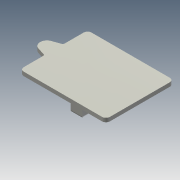
# Autodesk Inventor part: ball
Saved by Autodesk Inventor 2015 (Build 190159000, 159)
## iProperties
Created: 2017-05-03
Part Number: ball
Material: 일반
Document SubType Name: Modeling
Designer: gatew
Density: 1 g/cm^3
Appearance: 기본값
Author: gatew
Autodesk Inventor part; units mm, degrees
ref_plane "작업 평면3" through (0, 30.3443, 0) normal (0, 1, 0) x (1, 0, 0)
sketch "스케치5" plane through (0, 30.3443, 0) normal (0, 1, 0) x (1, 0, 0)
  line L0 (-35, -52.5) -> (35, -52.5)
  line L1 (35, -52.5) -> (35, 52.5)
  line L2 (35, 52.5) -> (-35, 52.5)
  line L3 (-35, 52.5) -> (-35, -52.5)
  line L4 (-35, -52.5) -> (35, 52.5) construction
  line L5 (35, -52.5) -> (-35, 52.5) construction
  point P0 (0, 0)
  dimension "d33" = 70
  dimension "d34" = 105
  constraints: 12 end point, 2 midpoint, 2 parallel, 1 horizontal, 1 perpendicular
  measures "d33" distance of L2.end L1.end
  measures "d34" distance of L1.end L0.end
extrude "돌출3" add sketch "스케치5" along normal blind 4
ref_plane "작업 평면4" through (0, 30.3443, 0) normal (0, -1, 0) x (1, 0, 0)
ref_plane "작업 평면1" through (0, 0, 0) normal (0, -0.7071068, 0.7071068) x (1, 0, 0)
ref_plane "작업 평면2" through (0, 17.1721, 0) normal (0, 1, 0) x (-1, 0, 0)
sketch "스케치9" plane through (0, 0, 0) normal (1, 0, 0) x (0, 1, 0)
  point P0 (0, 0)
sketch "스케치11" plane through (0, 0, 0) normal (1, 0, 0) x (0, 1, 0)
  arc A0 (7.4999, 0) -> (21.3443, -3.9998) centre (14.9999, 0) ccw
  line L0 (30.3443, -6) -> (30.3443, 6) projected
  line L1 (30.3443, -3.9998) -> (21.3443, -3.9998)
  line L2 (30.3014, 0) -> (7.4999, 0)
  line L3 (30.3014, 0) -> (30.3443, 0)
  line L4 (30.3443, 6) -> (30.3443, -6) projected
  line L5 (30.3443, 0) -> (30.3443, -3.9998)
  point P0 (0, 0)
  dimension "d73" = 15
  dimension "d74" = 4
  dimension "d75" = 9
  dimension "d76" = 0
  constraints: 8 end point, 2 horizontal, 2 point on circle, 2 point on line, 1 centre point, 1 midpoint
  measures "d73" diameter of A0
  measures "d74" distance of L2.start L1.start
  measures "d75" distance of L1.end L1.start
  measures "d76" vertical distance of point (0, 0) A0.centre
revolve "회전2" add sketch "스케치11" angle 360 about axis through (0, 30.3014, 0) along (0, -1, 0)
fillet "모깎기12" radius 4 4 edges at (-35, 32.3443, 52.5) (-35, 32.3443, -52.5) (35, 32.3443, -52.5) (35, 32.3443, 52.5)
sketch "스케치24" plane through (0, 30.3443, 0) normal (0, -1, 0) x (1, 0, 0)
  line L0 (6, 48.5) -> (-6, 48.5)
  line L1 (-6, 48.5) -> (-6, 38.5)
  line L2 (-6, 38.5) -> (6, 38.5)
  line L3 (6, 38.5) -> (6, 48.5)
  line L4 (6, 48.5) -> (-6, 38.5) construction
  line L5 (-6, 48.5) -> (6, 38.5) construction
  line L6 (-31, 52.5) -> (31, 52.5) projected
  line L7 (0, 0) -> (8.4615, 0)
  line L8 (0, 0) -> (0, 7.732)
  line L9 (29, 6) -> (19, 6)
  line L10 (19, 6) -> (19, -6)
  line L11 (19, -6) -> (29, -6)
  line L12 (29, -6) -> (29, 6)
  line L13 (29, 6) -> (19, -6) construction
  line L14 (19, 6) -> (29, -6) construction
  line L15 (35, 48.5) -> (35, -48.5) projected
  line L16 (-29, 6) -> (-19, 6)
  line L17 (-19, 6) -> (-19, -6)
  line L18 (-19, -6) -> (-29, -6)
  line L19 (-29, -6) -> (-29, 6)
  line L20 (-29, 6) -> (-19, -6) construction
  line L21 (-19, 6) -> (-29, -6) construction
  point P0 (0, 43.5)
  point P1 (-6.0892, 52.5)
  point P2 (24, 0)
  point P3 (-24, 0)
  dimension "d116" = 12
  dimension "d117" = 10
  dimension "d118" = 9
  dimension "d119" = 10
  dimension "d120" = 12
  dimension "d121" = 11
  constraints: 40 end point, 6 midpoint, 5 symmetric about line, 4 parallel, 3 horizontal, 2 perpendicular, 1 vertical
  measures "d116" distance of L2.end L1.end
  measures "d117" distance of L1.end L0.end
  measures "d118" distance from line of L6 point (0, 43.5)
  measures "d119" distance of L11.end L10.end
  measures "d120" distance of L10.end L9.end
  measures "d121" distance from line of L15 point (24, 0)
extrude "돌출15" add sketch "스케치24" along normal blind 14
fillet "모깎기22" radius 2 10 edges at (29, 16.3443, 0) (24, 16.3443, -6) (19, 23.3443, -6) (19, 23.3443, 6) (24, 16.3443, 6) (0, 16.3443, 48.5) (-6, 23.3443, 38.5) (-6, 16.3443, 43.5) (6, 16.3443, 43.5) (6, 23.3443, 38.5)
fillet "모깎기23" radius 2 11 edges at (0, 30.3443, 38.5) (5.4142, 30.3443, 39.0858) (6, 30.3443, 44.5) (-6, 30.3443, 44.5) (-5.4142, 30.3443, 39.0858) (0, 30.3443, 3.9998) (19, 30.3443, 0) (19.5858, 30.3443, -5.4142) (25, 30.3443, -6) (25, 30.3443, 6) (19.5858, 30.3443, 5.4142)
fillet "모깎기24" radius 4 3 edges at (5.4142, 16.9301, 39.0858) (-5.4142, 16.9301, 39.0858) (0, 16.3443, 38.5)
fillet "모깎기26" radius 2 3 edges at (19.5858, 16.9301, -5.4142) (19.5858, 16.9301, 5.4142) (19, 16.3443, 0)
fillet "모깎기27" radius 2 1 edges at (29, 30.3443, 0)
sketch "스케치26" plane through (0, 30.3443, 0) normal (0, -1, 0) x (1, 0, 0)
  circle A0 centre (0, -59.5) radius 5
  line L0 (31, -52.5) -> (-31, -52.5) projected
  arc A1 (-6.5918, -61.8553) -> (6.5918, -61.8553) centre (0, -59.5) ccw
  line L1 (-6.5918, -61.8553) -> (-9.9346, -52.5)
  line L2 (6.5918, -61.8553) -> (9.5074, -52.5)
  line L3 (-9.9346, -52.5) -> (9.5074, -52.5)
  point P0 (0, 0)
  dimension "d141" = 10
  dimension "d142" = 7
  dimension "d153" = 7
  constraints: 6 end point, 2 centre point, 2 point on circle, 1 coincident, 1 collinear, 1 point on line, 1 tangent
  measures "d141" diameter of A0
  measures "d142" distance from line of A0.centre L0
  measures "d153" radius of A1
extrude "돌출16" add sketch "스케치26" against normal up to surface (4 mm away) contours A0 | L2 A1 L1 L0
sketch "스케치27" plane through (0, 30.3443, 0) normal (0, -1, 0) x (1, 0, 0)
  circle A0 centre (0, -59.5) radius 5
  line L0 (31, -52.5) -> (9.5074, -52.5) projected
  point P0 (0, 0)
  dimension "d145" = 10
  dimension "d146" = 7
  constraints: 1 centre point
  measures "d145" diameter of A0
  measures "d146" distance from line of L0 A0.centre
extrude "돌출17" cut sketch "스케치27" against normal blind 3
fillet "모깎기28" radius 2 2 edges at (-9.9346, 32.3443, -52.5) (9.5074, 32.3443, -52.5)
sketch "스케치28" plane through (0, 33.3443, -59.5) normal (0, -1, 0) x (1, 0, 0)
  circle A0 centre (0, 0) radius 3.9
  point P0 (0, 59.5)
  dimension "d150" = 7.8
  constraints: 1 centre point
  measures "d150" diameter of A0
extrude "돌출18" add sketch "스케치28" along normal blind 9
mirror "대칭3" about plane through (0, 0, 0) normal (0, 0, 1) of "돌출16"
mirror "대칭4" about plane through (0, 0, 0) normal (0, 0, 1) of "돌출17"
mirror "대칭5" about plane through (0, 0, 0) normal (0, 0, 1) of "모깎기28"
mirror "대칭6" about plane through (0, 0, 0) normal (0, 0, 1) of "돌출18"
sketch "스케치29" plane through (-31, 30.3443, -52.5) normal (0, 0, -1) x (-1, 0, 0)
  line L0 (7.4469, -7.4919) -> (-69.4469, -7.4919)
  line L1 (-69.4469, -7.4919) -> (-69.4469, 12.0532)
  line L2 (-69.4469, 12.0532) -> (7.4469, 12.0532)
  line L3 (7.4469, 12.0532) -> (7.4469, -7.4919)
  line L4 (7.4469, -7.4919) -> (-69.4469, 12.0532) construction
  line L5 (-69.4469, -7.4919) -> (7.4469, 12.0532) construction
  point P0 (-31, -30.3443)
  point P1 (-31, 2.2807)
  constraints: 12 end point, 2 midpoint, 2 parallel, 1 horizontal, 1 perpendicular
extrude "돌출19" cut sketch "스케치29" against normal blind 20
extrude "돌출20" cut sketch "스케치29" along normal blind 20
sketch "스케치30" plane through (0, 30.3443, 0) normal (0, -1, 0) x (1, 0, 0)
  line L0 (35, -32.5) -> (-35, -32.5)
  line L1 (-35, -32.5) -> (-35, -32.5)
  line L2 (-31, -36.5) -> (31, -36.5)
  line L3 (35, -32.5) -> (35, -32.5)
  line L4 (35, -32.5) -> (-35, -32.5) projected
  arc A0 (31, -36.5) -> (35, -32.5) centre (31, -32.5) ccw
  arc A1 (-35, -32.5) -> (-31, -36.5) centre (-31, -32.5) ccw
  point P0 (0, 0)
  point P1 (-35, -36.5)
  dimension "d158" = 4
  dimension "d159" = 4
  constraints: 8 end point, 4 point on circle, 4 tangent, 3 perpendicular, 2 centre point, 2 point on line, 1 equal radius, 1 horizontal
  measures "d158" distance of L0.end point (-35, -36.5)
  measures "d159" radius of A0
extrude "돌출21" add sketch "스케치30" against normal up to surface (4 mm away)
fillet "모깎기29" radius 4 4 edges at (-19, 16.3443, 0) (-19, 23.3443, -6) (-19, 30.3443, 0) (-19, 23.3443, 6)
fillet "모깎기30" radius 2 5 edges at (-29, 16.3443, 0) (-20.1716, 17.5159, -4.8284) (-26, 16.3443, -6) (-20.1716, 17.5159, 4.8284) (-26, 16.3443, 6)
fillet "모깎기31" radius 2 1 edges at (-29, 30.3443, 0)
